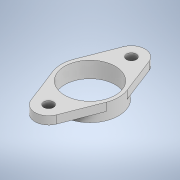
# Autodesk Inventor part: chumacera
Saved by Autodesk Inventor 2021 (Build 250183000, 183)
## iProperties
Created: 2021-04-05
Part Number: chumacera
Material: Generic
Document SubType Name: Modeling
Designer: jorge
Density: 1 g/cm^3
Appearance: Default
Author: jorge
Autodesk Inventor part; units mm, degrees
ref_plane "YZ Plane" through (0, 0, 0) normal (1, 0, 0) x (0, 1, 0)
ref_plane "XZ Plane" through (0, 0, 0) normal (0, 1, 0) x (-1, 0, 0)
ref_plane "XY Plane" through (0, 0, 0) normal (0, 0, 1) x (1, 0, 0)
sketch "Sketch1" plane through (0, 0, 0) normal (0, 1, 0) x (-1, 0, 0)
  circle A0 centre (0, 0) radius 11
  circle A1 centre (0, 0) radius 12.5
  dimension "d0" = 22
  dimension "d1" = 25
  constraints: 2 centre point, 2 coincident
  measures "d0" diameter of A0
  measures "d1" diameter of A1
extrude "Extrusion1" add sketch "Sketch1" along normal blind 7
sketch "Sketch2" plane through (0, 7, 0) normal (0, 1, 0) x (1, 0, 0)
  circle A0 centre (0, -18.05) radius 2.15
  circle A1 centre (0, 18.05) radius 2.15
  circle A2 centre (0, -18.05) radius 5.95
  circle A3 centre (0, 18.05) radius 5.95
  line L0 (-5.5444, -20.2091) -> (-11.6479, -4.536)
  line L1 (5.5444, -20.2091) -> (11.6479, -4.536)
  line L2 (-11.6479, 4.536) -> (-5.5444, 20.2091)
  line L3 (11.6479, 4.536) -> (5.5444, 20.2091)
  circle A4 centre (0, 0) radius 12.5 projected
  dimension "d4" = 4.3
  dimension "d5" = 4.3
  dimension "d6" = 0
  dimension "d7" = 0
  dimension "d8" = 18.05
  dimension "d9" = 18.05
  dimension "d10" = 3.8
  dimension "d11" = 3.8
  constraints: 8 end point, 8 point on circle, 8 tangent, 4 centre point
  measures "d4" diameter of A0
  measures "d5" diameter of A1
  measures "d6" horizontal distance of A1.centre point (0, 0)
  measures "d7" horizontal distance of point (0, 0) A0.centre
  measures "d8" distance of A1.centre point (0, 0)
  measures "d9" distance of A0.centre point (0, 0)
  measures "d10" radial gap between concentric circles of A0 A2
  measures "d11" radial gap between concentric circles of A1 A3
extrude "Extrusion2" add sketch "Sketch2" against normal blind 3.5 contours A2 A4 | L0 A4 A2 | A2 A4 L1 | L2 A3 A4 | A3 A4 | A4 A3 L3 picked at (3.4679, -21.155) picked at (3.4679, 21.155)
body "Solid1"
